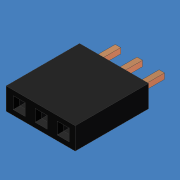
# Autodesk Inventor part: 1x3 Header Connector
Saved by Autodesk Inventor 2012 (Build 160160000, 160)
## iProperties
Shininess: 64.0
Length Units: 11272
Angle Units: 11279
Time Units: 11290
Mass Units: 11286
Length Display Precision: 3
Angle Display Precision: 2
Compacted: True
Part Number: 1x3 Header Connector
Document SubType Name: Modeling
Created: 2006-01-04
Designer: Owner
Material: ABS Plastic
Density: 1 g/cm^3
Density: 0.0
Volumn: 0.0
Area: 0.0
PropertySet Name: Model Information
Control State: 0
Master: False
Checked Out: False
Author: Owner
Autodesk Inventor part; units mm, degrees
ref_plane "YZ Plane" through (0, 0, 0) normal (1, 0, 0) x (0, 1, 0)
ref_plane "XZ Plane" through (0, 0, 0) normal (0, 1, 0) x (-1, 0, 0)
ref_plane "XY Plane" through (0, 0, 0) normal (0, 0, 1) x (1, 0, 0)
sketch "Sketch1" plane through (0, 0, 0) normal (0, 0, 1) x (1, 0, 0)
  line L0 (-4.0005, 1.27) -> (4.0005, 1.27)
  line L1 (4.0005, 1.27) -> (4.0005, -1.27)
  line L2 (4.0005, -1.27) -> (-4.0005, -1.27)
  line L3 (-4.0005, -1.27) -> (-4.0005, 1.27)
  line L4 (0, 0) -> (-4.0005, 0) construction
  line L5 (0, 0) -> (0, -1.27) construction
  line L6 (0, 0) -> (0, 1.27) construction
  line L7 (0, 0) -> (4.0005, 0) construction
  dimension "d0" = 8.001
  dimension "d1" = 2.54
  constraints: 16 end point, 4 midpoint, 3 horizontal, 2 collinear, 2 parallel, 2 vertical, 1 perpendicular, 1 other
  measures "d0" distance of L0.start L0.end
  measures "d1" distance of L0.end L1.end
extrude "Extrusion1" add sketch "Sketch1" along normal blind 8.509
sketch "Sketch2" plane through (0, 0, 8.509) normal (0, 0, 1) x (1, 0, 0)
  line L0 (-4.0005, 1.27) -> (4.0005, 1.27) projected
  line L1 (-4.0005, -1.27) -> (-4.0005, 1.27) projected
  line L2 (-2.794, 0.3175) -> (-2.159, 0.3175)
  line L3 (-2.159, 0.3175) -> (-2.159, -0.3175)
  line L4 (-2.159, -0.3175) -> (-2.794, -0.3175)
  line L5 (-2.794, -0.3175) -> (-2.794, 0.3175)
  dimension "d4" = 0.635
  dimension "d5" = 1.2065
  dimension "d6" = 0.9525
  constraints: 8 end point, 2 parallel, 2 perpendicular, 1 horizontal
  measures "d4" distance of L2.start L2.end
  measures "d5" distance between parallel lines of L1 L5
  measures "d6" distance between parallel lines of L0 L2
extrude "Extrusion2" cut sketch "Sketch2" against normal blind 6.35
chamfer "Chamfer1" distance 0.381 angle 45 4 edges at (-2.4765, 0.3175, 8.509) (-2.159, 0, 8.509) (-2.4765, -0.3175, 8.509) (-2.794, 0, 8.509)
sketch "Sketch3" plane through (0, 0, 2.159) normal (0, 0, 1) x (1, 0, 0)
  line L0 (-2.794, 0.3175) -> (-2.794, -0.3175) projected
  line L1 (-2.794, -0.3175) -> (-2.794, 0.3175) projected
  line L2 (-2.794, 0.3175) -> (-2.159, 0.3175) projected
  line L3 (-2.159, 0.3175) -> (-2.159, -0.3175) projected
  line L4 (-2.159, -0.3175) -> (-2.794, -0.3175) projected
extrude "Extrusion3" add sketch "Sketch3" against normal blind 5.08
pattern_linear "Rectangular Pattern3" count 3 spacing 2.54 along (1, 0, 0) of "Extrusion2", "Chamfer1"
pattern_linear "Rectangular Pattern4" count 3 spacing 2.54 along (1, 0, 0) of "Extrusion3"
body "Solid1"
